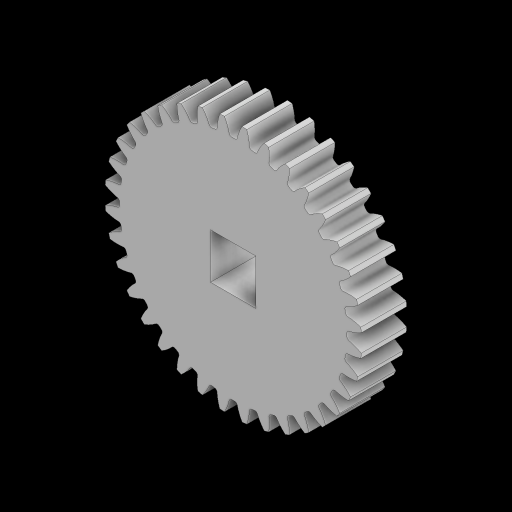
# Autodesk Inventor part: OutPutGear
Saved by Autodesk Inventor 2024.1 (Build 281209000, 209)
## iProperties
Created: 2025-02-21
Part Number: OutPutGear
Material: Generic
Document SubType Name: Modeling
Designer: Teddy
Density: 1 g/cm^3
Appearance: Default
Author: Teddy
Autodesk Inventor part; units mm, degrees
ref_plane "YZ Plane" through (0, 0, 0) normal (1, 0, 0) x (0, 1, 0)
ref_plane "XZ Plane" through (0, 0, 0) normal (0, 1, 0) x (-1, 0, 0)
ref_plane "XY Plane" through (0, 0, 0) normal (0, 0, 1) x (1, 0, 0)
sketch "Sketch1" plane through (0, 0, 0) normal (0, 0, 1) x (1, 0, 0)
  spline S0 degree 3 poles (-1.2344, 17.9031) (-1.1833, 17.8096) (-1.0809, 17.6225) (-0.9666, 17.3814) (-0.8822, 17.1856) (-0.823, 17.037) (-0.7683, 16.8867) (-0.7186, 16.7346) (-0.6749, 16.5807) (-0.6373, 16.4252) (-0.6161, 16.2934) (-0.5849, 16.1912) (-0.5522, 16.1182) (-0.5104, 16.0496) (-0.4565, 15.99) (-0.392, 15.9419) (-0.3309, 15.9142) (-0.2795, 15.8997) (-0.2267, 15.8919) (-0.1332, 15.8924) (0, 15.8937) (0.1332, 15.8924) (0.2267, 15.8919) (0.2795, 15.8997) (0.3309, 15.9142) (0.392, 15.9419) (0.4565, 15.99) (0.5104, 16.0496) (0.5522, 16.1182) (0.5849, 16.1912) (0.6161, 16.2934) (0.6373, 16.4252) (0.6749, 16.5807) (0.7186, 16.7346) (0.7683, 16.8867) (0.823, 17.037) (0.8822, 17.1856) (0.9666, 17.3814) (1.0809, 17.6225) (1.1833, 17.8096) (1.2344, 17.9031) knots 0 0 0 0 0.031987 0.063974 0.079968 0.095962 0.111957 0.127951 0.143944 0.159938 0.175929 0.183922 0.191911 0.199899 0.207889 0.215879 0.223867 0.227865 0.231863 0.239856 0.255849 0.271842 0.279835 0.283833 0.287831 0.295819 0.303809 0.311799 0.319787 0.327776 0.335769 0.351761 0.367754 0.383748 0.399742 0.415736 0.43173 0.447725 0.479711 0.511698 0.511698 0.511698 0.511698
  circle A0 centre (0, 0) radius 15.8932 construction
  circle A1 centre (0, 0) radius 16.2132 construction
  circle A2 centre (0, 0) radius 17 construction
  circle A3 centre (0, 0) radius 17.9456
  point P0 (-1.0836, 17.621)
  point P1 (-0.9461, 17.3322)
  point P2 (-0.8829, 17.1853)
  point P3 (-0.8237, 17.0367)
  point P4 (-0.7691, 16.8864)
  point P5 (-0.7196, 16.7343)
  point P6 (-0.6759, 16.5804)
  point P7 (-0.6393, 16.4248)
  point P8 (-0.6071, 16.2681)
  point P9 (-0.5834, 16.1918)
  point P10 (-0.5507, 16.1189)
  point P11 (-0.5084, 16.0511)
  point P12 (-0.4548, 15.9919)
  point P13 (-0.3905, 15.9444)
  point P14 (-0.3179, 15.9112)
  point P15 (-0.2793, 15.9005)
  point P16 (-0.2398, 15.8945)
  point P17 (-0.1599, 15.8923)
  point P18 (0, 15.8932)
  point P19 (0.1599, 15.8923)
  point P20 (0.2398, 15.8945)
  point P21 (0.2793, 15.9005)
  point P22 (0.3179, 15.9112)
  point P23 (0.3905, 15.9444)
  point P24 (0.4548, 15.9919)
  point P25 (0.5084, 16.0511)
  point P26 (0.5507, 16.1189)
  point P27 (0.5834, 16.1918)
  point P28 (0.6071, 16.2681)
  point P29 (0.6393, 16.4248)
  point P30 (0.6759, 16.5804)
  point P31 (0.7196, 16.7343)
  point P32 (0.7691, 16.8864)
  point P33 (0.8237, 17.0367)
  point P34 (0.8829, 17.1853)
  point P35 (0.9461, 17.3322)
  point P36 (1.0836, 17.621)
  dimension "d11" = 34.0106
  constraints: 4 centre point, 2 point on circle, 83 other
extrude "Extrusion1" add sketch "Sketch1" against normal blind 6.35
extrude "Extrusion2" cut sketch "Sketch1" against normal blind 25.4 contours A3 S0 picked at (-0.1045, 17.1735)
pattern_circular "Circular Pattern1" count 36 over 360 about axis through (0, 0, 0) along (0, 0, -1) of "Extrusion2"
sketch "Sketch2" plane through (0, 0, 0) normal (0, 0, 1) x (1, 0, 0)
  line L0 (-3.175, -3.175) -> (3.175, -3.175)
  line L1 (3.175, -3.175) -> (3.175, 3.175)
  line L2 (3.175, 3.175) -> (-3.175, 3.175)
  line L3 (-3.175, 3.175) -> (-3.175, -3.175)
  line L4 (-3.175, -3.175) -> (3.175, 3.175) construction
  line L5 (3.175, -3.175) -> (-3.175, 3.175) construction
  point P0 (0, 0)
  dimension "d7" = 6.35
  dimension "d8" = 6.35
  constraints: 12 end point, 2 midpoint, 2 parallel, 1 horizontal, 1 perpendicular
  measures "d7" distance of L2.end L1.end
  measures "d8" distance between parallel lines of L2 L0
extrude "Extrusion3" cut sketch "Sketch2" against normal blind 6.35
equation "\"Module\" = 1"
equation "\"PressureAngle\" = 17.5deg"
equation "\"UnitProfileAddendum\" = 0.8"
equation "\"UnitProfileClearance\" = 0.25"
equation "\"UnitRoundRadius\" = 0.3335"
equation "\"HeadDiameter\" = 35.89126"
equation "\"RootDiameter\" = 31.7864"
equation "\"BaseDiameter\" = 32.42638"
equation "\"PitchDiameter\" = 34"
equation "\"FaceWidth\" = 3.81"
equation "\"HelixAngle\" = 0"
equation "\"UnitCorrection\" = 0.154371"
equation "\"UnitAddendumModification\" = 0.008742"
equation "\"CircularPitch\" = 3.141593"
equation "\"UnitBacklashShift\" = -0.21117"
equation "\"TotalToolShift\" = -0.0568"
equation "\"IsInternal\" = 0"
body "Solid1"
